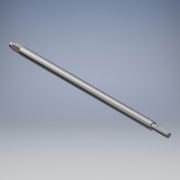
# Autodesk Inventor part: Saftey Axle
Saved by Autodesk Inventor 2019.4 (Build 234330000, 330)
## iProperties
Created: 2020-01-29
Part Number: Saftey Axle
Material: Steel, Alloy
Document SubType Name: Modeling
Designer: admin
Density: 7.73 g/cm^3
Appearance: Semi-Polished
Mass: 223.395 g
Surface Area: 102.772 cm^2
Volume: 28.8997 cm^3
Author: admin
Autodesk Inventor part; units mm, degrees
ref_plane "YZ Plane" through (0, 0, 0) normal (1, 0, 0) x (0, 1, 0)
ref_plane "XZ Plane" through (0, 0, 0) normal (0, 1, 0) x (-1, 0, 0)
ref_plane "XY Plane" through (0, 0, 0) normal (0, 0, 1) x (1, 0, 0)
sketch "Sketch1" plane through (0, 0, 0) normal (0, 0, 1) x (1, 0, 0)
  line L0 (0, 0) -> (0, 4)
  line L1 (0, 4) -> (4, 4)
  line L2 (4, 4) -> (4, 6)
  line L3 (4, 6) -> (250.6, 6)
  line L4 (250.6, 6) -> (250.6, 4)
  line L5 (250.6, 4) -> (258.6, 4)
  line L6 (258.6, 4) -> (258.6, 3.75)
  line L7 (258.6, 3.75) -> (259.7, 3.75)
  line L8 (259.7, 3.75) -> (259.7, 4)
  line L9 (259.7, 4) -> (275.7, 4)
  line L10 (275.7, 4) -> (275.7, 3.75)
  line L11 (275.7, 3.75) -> (276.8, 3.75)
  line L12 (276.8, 3.75) -> (276.8, 4)
  line L13 (276.8, 4) -> (278.8, 4)
  line L14 (278.8, 4) -> (278.8, 0)
  line L15 (278.8, 0) -> (0, 0)
  dimension "d0" = 4
  dimension "d1" = 4
  dimension "d2" = 6
  dimension "d3" = 1.1
  dimension "d4" = 1.1
  dimension "d5" = 0.25
  dimension "d6" = 2
  dimension "d7" = 16
  dimension "d8" = 246.6
  dimension "d9" = 8
  constraints: 32 end point, 11 perpendicular, 8 point on line, 1 vertical
  measures "d0" distance of L0.end L1.end
  measures "d1" distance between parallel lines of L15 L1
  measures "d2" distance between parallel lines of L15 L3
  measures "d3" distance of L6.end L7.end
  measures "d4" distance of L10.end L11.end
  measures "d5" distance of L5.end L6.end
  measures "d6" distance of L12.end L13.end
  measures "d7" distance of L8.end L9.end
  measures "d8" distance of L2.end L3.end
  measures "d9" distance of L4.end L5.end
revolve "Revolution1" add sketch "Sketch1" angle 360 about axis through (278.8, 0, 0) along (-1, 0, 0)
sketch "Sketch2" plane through (278.8, 0, 0) normal (1, 0, 0) x (0, 0, -1)
  line L0 (-2.6458, 3) -> (2.6458, 3)
  circle A0 centre (0, 0) radius 4 projected
  point P0 (0, 0)
  dimension "d11" = 3
  constraints: 2 end point, 2 point on circle, 1 horizontal
  measures "d11" distance from line of point (0, 0) L0
extrude "Extrusion1" cut sketch "Sketch2" against normal up to surface (20.2 mm away) contours A0 L0 picked at (-0.6179, 3.1815)
sketch "Sketch4" plane through (4, 0, 0) normal (-1, 0, 0) x (0, 0, 1)
  line L0 (2.7496, 4.7625) -> (5.4993, 0)
  line L1 (5.4993, 0) -> (2.7496, -4.7625)
  line L2 (2.7496, -4.7625) -> (-2.7496, -4.7625)
  line L3 (-2.7496, -4.7625) -> (-5.4993, 0)
  line L4 (-5.4993, 0) -> (-2.7496, 4.7625)
  line L5 (-2.7496, 4.7625) -> (2.7496, 4.7625)
  line L6 (0, 4.7625) -> (0, 0) construction
  circle A0 centre (0, 0) radius 6.5
  dimension "d19" = 9.525
  dimension "d20" = 13
  constraints: 14 end point, 2 coincident, 1 centre point, 1 midpoint, 1 vertical, 13 other
  measures "d19" distance between parallel lines of L2 L5
  measures "d20" diameter of A0
extrude "Extrusion3" cut sketch "Sketch4" against normal blind 15
ref_plane "Work Plane1" through (6, 0, 0) normal (-1, 0, 0) x (0, 0, 1)
sketch "Sketch6" plane through (6, 0, 0) normal (-1, 0, 0) x (0, 0, 1)
  circle A0 centre (0, 0) radius 4.8
  circle A1 centre (0, 0) radius 12.5
  dimension "d27" = 9.6
  dimension "d28" = 25
  constraints: 2 centre point, 2 coincident
  measures "d27" diameter of A0
  measures "d28" diameter of A1
extrude "Extrusion5" cut sketch "Sketch6" along normal blind 1.1
body "Solid1"
